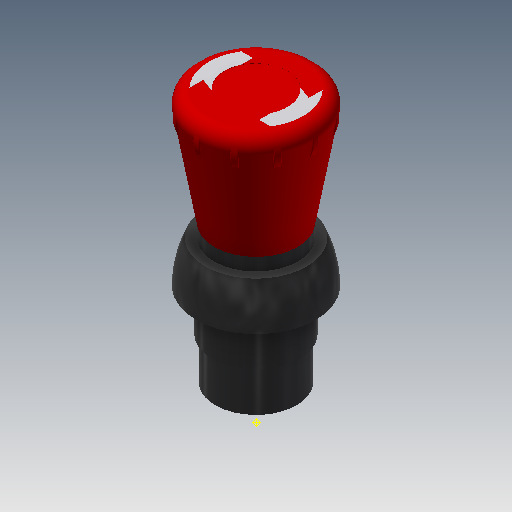
# Autodesk Inventor part: 800MR-D1D1
Saved by Autodesk Inventor 2019.1 (Build 231200000, 200)
## iProperties
Created: 2005-06-20
Part Number: 800MR-D1D1
Checked By: ~
Material: Delrin, Black
Document SubType Name: Modeling
Designer: BASSBW
Manufacturer: Standard
Standards Organization: Custom
Density: 1.425 g/cm^3
Appearance: Dark Gray
Description: PUSH BUTTON - MUSHROOM, NEMA 13
Vendor: AB
GlobalPropertyList: <PropertyList/>
Application ID: AutoCAD Electrical
Category: PB
SCALE: 1:1
STOCK SIZE: SEE DWG
UNITS: ANSI
COMMODITY: MFG
Author: BassBW
Autodesk Inventor part; units mm, degrees
ref_plane "YZ Plane" through (0, 0, 0) normal (1, 0, 0) x (0, 1, 0)
ref_plane "XZ Plane" through (0, 0, 0) normal (0, 1, 0) x (-1, 0, 0)
ref_plane "XY Plane" through (0, 0, 0) normal (0, 0, 1) x (1, 0, 0)
sketch "Sketch9" plane through (0, 0, 0) normal (0, 0, 1) x (1, 0, 0)
  line L0 (0, 0) -> (0, 10.5)
  line L1 (0, 0) -> (15, 0)
  arc A0 (15, 0) -> (12.728121, 10.5) centre (-10.4, 0) ccw
  line L2 (12.728121, 10.5) -> (0, 10.5)
  dimension "d35" = 30
  dimension "d37" = 25.4
  dimension "d43" = 10.5
  constraints: 6 end point, 2 perpendicular, 2 point on circle, 1 centre point, 1 point on line, 1 vertical
  measures "d35" diameter of L1.end L0
  measures "d37" radius of A0
  measures "d43" distance between parallel lines of L2 L1
revolve "Revolution1" add sketch "Sketch9" angle 360 about axis through (0, 0, 0) along (0, 1, 0)
sketch "Sketch10" plane through (0, 10.5, 0) normal (0, 1, 0) x (1, 0, 0)
  circle A0 centre (0, 0) radius 12.728121
  circle A1 centre (0, 0) radius 10.5
  dimension "d39" = 21
  constraints: 1 centre point, 1 coincident
  measures "d39" diameter of A1
extrude "Extrusion6" add sketch "Sketch10" along normal blind 3.175 contours A1
sketch "Sketch11" plane through (0, 0, 0) normal (0, -1, 0) x (1, 0, 0)
  circle A0 centre (0, 0) radius 15 projected
  circle A1 centre (0, 0) radius 11
  circle A2 centre (0, 0) radius 7.9375
  dimension "d42" = 22
  dimension "d44" = 15.875
  constraints: 2 centre point, 2 coincident
  measures "d42" diameter of A1
  measures "d44" diameter of A2
extrude "Extrusion7" add sketch "Sketch11" along normal blind 10.5 contours A1
sketch "Sketch12" plane through (0, -10.5, 0) normal (0, -1, 0) x (1, 0, 0)
  circle A0 centre (0, 0) radius 7.9375 projected
  circle A1 centre (0, 0) radius 11 projected
  circle A2 centre (0, 0) radius 10.2108
  dimension "d47" = 20.4216
  constraints: 1 centre point, 1 coincident
  measures "d47" diameter of A2
extrude "Extrusion8" add sketch "Sketch12" along normal blind 10.5 contours A2
sketch "Sketch13" plane through (0, 13.675, 0) normal (0, 1, 0) x (1, 0, 0)
  circle A0 centre (0, 0) radius 10.5 projected
extrude "Extrusion9" add sketch "Sketch13" along normal blind 29.21 draft 10
fillet "Fillet1" radius 3.175 1 edges at (-15.6505, 42.885, 0)
sketch "Sketch15" plane through (0, 42.885, 0) normal (0, 1, 0) x (1, 0, 0)
  circle A0 centre (0, 0) radius 11.866693
  circle A1 centre (0, 0) radius 7.9375
  dimension "d53" = 15.875
  constraints: 1 centre point, 1 coincident
  measures "d53" diameter of A1
extrude "Extrusion10" cut sketch "Sketch15" against normal blind 0.0254 contours A1
sketch "Sketch16" plane through (0, 42.885, 0) normal (0, 1, 0) x (1, 0, 0)
  circle A0 centre (0, 0) radius 7.9375
  circle A1 centre (0, 0) radius 11.866693
  line L0 (-7.140776, 3.466011) -> (-7.140776, 6.35)
  line L1 (-7.140776, 6.35) -> (-10.024765, 6.35)
  line L2 (-5.340244, -5.872453) -> (-8.612398, -4.681486)
  line L3 (-8.612398, -4.681486) -> (-8.612398, -8.16364)
  dimension "d57" = 6.35
  dimension "d59" = 70
  dimension "d60" = 8.6124
  constraints: 8 end point, 4 point on circle, 2 equal length, 2 perpendicular, 1 vertical
  measures "d57" distance from line of A0.centre L1
  measures "d59" angle of L3 L2
  measures "d60" distance from line of L3 A0.centre
extrude "Extrusion11" add sketch "Sketch16" along normal blind 0.0254 contours A0 L2 L3 A1 L1 L0 picked at (-10.292742, -2.119141)
pattern_circular "Circular Pattern1" count 2 over 360 about axis through (0, 13.675, 0) along (0, 1, 0) of "Extrusion11"
sketch "Sketch17" plane through (0, 0, 0) normal (1, 0, 0) x (0, 1, 0)
  line L0 (13.675, 10.5) -> (13.675, -10.5)
  line L1 (39.158667, -14.993458) -> (39.158667, 14.993458)
  arc A0 (42.885, 11.866693) -> (39.158667, 14.993458) centre (39.71, 11.866693) ccw
  line L2 (13.675, 10.5) -> (39.158667, 14.993458)
  arc A1 (40.261333, 14.993458) -> (35.452734, 14.340002) centre (38.761792, 8.008865) ccw
  line L3 (-27.461402, 0) -> (62.998222, 0)
  dimension "d66" = 7.14375
  dimension "d67" = 0.39687
  dimension "d71" = 8.00886
  constraints: 3 point on circle, 1 centre point, 1 point on line
  measures "d66" radius of A1
  measures "d67" distance from line of A1.centre L1
  measures "d71" distance from line of L3 A1.centre
extrude "Extrusion12" add sketch "Sketch17" along normal mid plane 1.5875 contours A1 A0 L2
fillet "Fillet2" radius 0.254 1 edges at (0.7937, 37.7998, 15.0876)
fillet "Fillet3" radius 0.254 1 edges at (-0.7937, 37.7998, 15.0876)
pattern_circular "Circular Pattern2" count 12 over 360 about axis through (0, 13.675, 0) along (0, 1, 0) of "Extrusion12", "Fillet2", "Fillet3"
sketch "Sketch18" plane through (0, -21, 0) normal (0, -1, 0) x (1, 0, 0)
  circle A0 centre (0, 0) radius 5
  point P0 (0, 5)
  point P1 (0, -5)
  dimension "d78" = 10
  constraints: 2 point on circle, 1 centre point, 1 coincident
  measures "d78" diameter of A0
equation "\"d57\" = d56"
equation "\"d56\" = 6.35"
body "Solid1"
